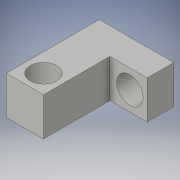
# Autodesk Inventor part: Pivot Point 2
Saved by Autodesk Inventor 2016 (Build 200138000, 138)
## iProperties
Created: 2016-03-19
Part Number: Pivot Point 2
Material: Generic
Document SubType Name: Modeling
Designer: matth_000
Density: 1 g/cm^3
Appearance: Default
Author: matth_000
Autodesk Inventor part; units mm, degrees
ref_plane "YZ Plane" through (0, 0, 0) normal (1, 0, 0) x (0, 1, 0)
ref_plane "XZ Plane" through (0, 0, 0) normal (0, 1, 0) x (-1, 0, 0)
ref_plane "XY Plane" through (0, 0, 0) normal (0, 0, 1) x (1, 0, 0)
sketch "Sketch1" plane through (0, 0, 0) normal (0, 1, 0) x (-1, 0, 0)
  line L0 (0, 0) -> (-17.78, 0)
  line L1 (-17.78, 0) -> (-17.78, -44.45)
  line L2 (-17.78, -44.45) -> (0, -44.45)
  line L3 (0, -44.45) -> (0, 0)
  line L4 (-17.78, -44.45) -> (-35.56, -44.45)
  line L5 (-35.56, -44.45) -> (-35.56, -31.75)
  line L6 (-35.56, -31.75) -> (-17.78, -31.75)
  line L7 (-17.78, -31.75) -> (-17.78, -44.45)
  dimension "d0" = 17.78
  dimension "d1" = 44.45
  dimension "d2" = 17.78
  dimension "d3" = 12.7
  constraints: 16 end point, 4 parallel, 2 horizontal, 2 perpendicular
  measures "d0" distance of L2.end L1.end
  measures "d1" distance of L1.end L0.end
  measures "d2" distance of L5.end L6.end
  measures "d3" distance of L4.end L5.end
extrude "Extrusion1" add sketch "Sketch1" along normal blind 18.288
sketch "Sketch2" plane through (17.78, 0, -31.75) normal (0, 0, 1) x (1, 0, 0)
  circle A0 centre (9.4883, 9.144) radius 6.35
  point P0 (-17.78, 0)
  dimension "d6" = 12.7
  constraints: 1 centre point
  measures "d6" diameter of A0
extrude "Extrusion2" cut sketch "Sketch2" against normal blind 12.7
sketch "Sketch3" plane through (0, 18.288, 0) normal (0, 1, 0) x (1, 0, 0)
  circle A0 centre (8.89, 8.89) radius 6.35
  line L0 (0, 0) -> (17.78, 0) projected
  dimension "d9" = 12.7
  dimension "d10" = 8.89
  constraints: 1 centre point
  measures "d9" diameter of A0
  measures "d10" distance from line of L0 A0.centre
extrude "Extrusion3" cut sketch "Sketch3" against normal blind 18.288
body "Solid1"
